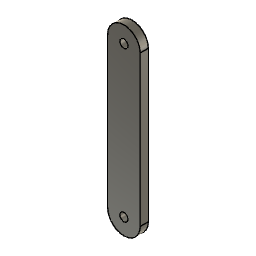
Brazo 2 Nueva Versión v5 (Autodesk Fusion 360 design; units mm, degrees)
Autodesk Fusion 360 part; units mm, degrees
sketch "Boceto1" plane through (0, 0, 0) normal (0, 1, 0) x (1, 0, 0)
  circle A0 centre (0, 0) radius 8
  circle A1 centre (0, 0) radius 10
  line L0 (-10, 0) -> (-10, -0.5331)
  line L1 (-10, -0.5331) -> (-10, -92.5331)
  line L2 (-10, -92.5331) -> (10, -92.5331)
  line L3 (10, -92.5331) -> (10, 0)
  circle A2 centre (0, -92.5331) radius 10
  dimension "d1" = 16
  dimension "d5" = 92
  constraint coincident A0.centre A1.centre
  constraint concentric A0 A1
  constraint coincident A1 L0.start
  constraint tangent A1 L0
  constraint vertical L0
  constraint parallel L0 L1
  constraint perpendicular L1 L2
  constraint coincident A1 L3.end
  constraint tangent A1 L3
  constraint perpendicular L2 L3
  constraint midpoint L2 A2.centre
  constraint coincident L1.end A2
  measures "d1" diameter of A0
  measures "d5" distance of L0.end L1.end
extrude "Extruir1" add sketch "Boceto1" along normal blind 5 makes body 1
sketch "Boceto2" plane through (0, 0, 0) normal (0, -1, 0) x (1, 0, 0)
  circle A0 centre (0, 0) radius 8
  line L0 (-10, 92.5331) -> (-10, 0)
  arc A1 (-10, 0) -> (10, 0) centre (0, 0) ccw
  line L1 (10, 0) -> (10, 92.5331)
  arc A2 (10, 92.5331) -> (-10, 92.5331) centre (0, 92.5331) ccw
  circle A3 centre (0, 92.5331) radius 2.5
  dimension "d6" = 5
  constraint concentric A2 A3
  measures "d6" diameter of A3
extrude "Extruir2" cut sketch "Boceto2" against normal blind 16 contours A3 bodies 1
ref_plane "PlanoDeObra1" through (0, 1.4375, -10) normal (0, 0, -1) x (1, 0, 0)
ref_plane "PlanoDeObra2" through (0, 3.4729, 102.5331) normal (0, 0, 1) x (-1, 0, 0)
sketch "Boceto3" plane through (0, 0, 0) normal (0, -1, 0) x (1, 0, 0)
  circle A0 centre (0, 92.5331) radius 2.5
  circle A1 centre (0, 0) radius 8
  line L0 (-10, 92.5331) -> (-10, 0)
  arc A2 (-10, 0) -> (10, 0) centre (0, 0) ccw
  line L1 (10, 0) -> (10, 92.5331)
  arc A3 (10, 92.5331) -> (-10, 92.5331) centre (0, 92.5331) ccw
  circle A4 centre (0, 0) radius 2.5
  circle A5 centre (0, 92.5331) radius 2.5
  dimension "d11" = 5
  dimension "d12" = 5
  constraint concentric A1 A4
  constraint concentric A0 A5
  measures "d11" diameter of A4
  measures "d12" diameter of A5
extrude "Extruir3" add sketch "Boceto3" against normal up to surface (5 mm away) contours A0 A5 bodies 1
extrude "Extruir4" add sketch "Boceto3" against normal up to surface (5 mm away) contours A1 bodies 1
extrude "Extruir5" cut sketch "Boceto3" against normal up to surface (5 mm away) contours A0 A5 bodies 1
sketch "Boceto4" plane through (0, 0, 0) normal (0, -1, 0) x (1, 0, 0)
  circle A0 centre (0, 92.5331) radius 2.5
  circle A1 centre (0, 0) radius 2.5
  line L0 (-10, 92.5331) -> (-10, 0)
  arc A2 (-10, 0) -> (10, 0) centre (0, 0) ccw
  line L1 (10, 0) -> (10, 92.5331)
  arc A3 (10, 92.5331) -> (-10, 92.5331) centre (0, 92.5331) ccw
  circle A4 centre (0, 92.5331) radius 2.65
  line L2 (11, 0) -> (11, 92.5331)
  arc A5 (11, 92.5331) -> (-11, 92.5331) centre (0, 92.5331) ccw
  line L3 (-11, 92.5331) -> (-11, 0)
  arc A6 (-11, 0) -> (11, 0) centre (0, 0) ccw
  line L4 (11, 92.5331) -> (11, 72.5331)
  line L5 (11, 72.5331) -> (-11, 72.5331)
  dimension "d19" = 5.3
  dimension "d20" = 1
  dimension "d21" = 20
  constraint concentric A0 A4
  constraint parallel L2 L4
  constraint coincident L3 L5.end
  constraint perpendicular L3 L5
  measures "d19" diameter of A4
  measures "d21" distance of L2.end L4.end
extrude "Extruir6" add sketch "Boceto4" against normal up to surface (5 mm away) separate body contours L0 L1 A3 L2 A5 L3 L4 L5 makes body 2
extrude "Extruir7" add sketch "Boceto4" along normal blind 10 contours L0 L1 A3 L5 | L0 L1 A3 L2 A5 L3 L4 L5 bodies 2
move_face "CarasDesfase1" offset -0.25 3 faces at (-7.6604, 3.3333, 98.961) (10, 1.6667, 79.1998) (-10, 1.6667, 85.8664) on bodies 2
hidden bodies 2
